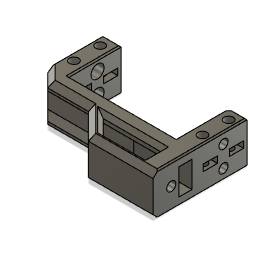
FrameAssembly v35 (Autodesk Fusion 360 archive; units mm, degrees)
design "FrameCenterServoHolder"
Autodesk Fusion 360 part; units mm, degrees
(part 1 of 2)
sketch "Sketch1" plane through (0, 0, 0) normal (0, 1, 0) x (1, 0, 0)
  line L0 (0, 26) -> (7, 26)
  line L1 (7, 26) -> (7, 6)
  line L2 (7, 6) -> (48, 6)
  line L3 (48, 6) -> (48, 26)
  line L4 (48, 26) -> (55, 26)
  line L5 (55, 26) -> (55, -9.8)
  line L6 (55, -9.8) -> (30.3, -9.8)
  line L7 (30.3, -9.8) -> (20.5, 0)
  line L8 (20.5, 0) -> (0, 0)
  line L9 (0, 26) -> (0, 0)
  line L10 (0, 0) -> (0, 39.3629) construction
  dimension "d1" = 7
  dimension "d2" = 7
  dimension "d3" = 41
  dimension "d4" = 6
  dimension "d5" = 15.8
  dimension "d7" = 135
  dimension "d8" = 20
  dimension "d98" = 20.5
  constraint perpendicular L0 L1
  constraint perpendicular L1 L2
  constraint perpendicular L2 L3
  constraint perpendicular L1 L4
  constraint perpendicular L4 L5
  constraint perpendicular L5 L6
  constraint collinear L0 L4
  constraint coincident L9.end L8
  constraint coincident L8.end L9.end
  constraint perpendicular L8 L9
  constraint vertical L10
  constraint collinear L9 L10
  measures "d1" distance of L0.start L0.end
  measures "d2" distance of L3.end L4.end
  measures "d3" distance of L1 L3
  measures "d4" distance of L2 L8
  measures "d5" distance of L2 L6
  measures "d7" angle of L6 L7
  measures "d8" distance of L2 L4
  measures "d98" distance of L7.end L8.end
extrude "Extrude1" add sketch "Sketch1" along normal blind 16
sketch "Sketch2" plane through (0, 16, 0) normal (0, 1, 0) x (-1, 0, 0)
  line L0 (-7, -26) -> (0, -26)
  line L1 (0, -26) -> (0, 0)
  line L2 (0, 0) -> (-20.5, 0)
  line L3 (-20.5, 0) -> (-30.3, 9.8)
  line L4 (-30.3, 9.8) -> (-55, 9.8)
  line L5 (-55, 9.8) -> (-55, -26)
  line L6 (-55, -26) -> (-48, -26)
  line L7 (-48, -26) -> (-48, -6)
  line L8 (-48, -6) -> (-7, -6)
  line L9 (-7, -6) -> (-7, -26)
  line L10 (-3, -22) -> (-52, -22) construction
  line L11 (-52, -22) -> (-52, -12) construction
  line L12 (-52, -12) -> (-3, -12) construction
  line L13 (-3, -12) -> (-3, -22) construction
  circle A0 centre (-3, -22) radius 1.75
  circle A1 centre (-3, -12) radius 1.75
  circle A2 centre (-52, -22) radius 1.75
  circle A3 centre (-52, -12) radius 1.75
  dimension "d11" = 3.5
  dimension "d12" = 3.5
  dimension "d13" = 3.5
  dimension "d14" = 3.5
  dimension "d15" = 49
  dimension "d16" = 10
  dimension "d17" = 55
  dimension "d18" = 20
  dimension "d19" = 4
  dimension "d20" = 3
  constraint horizontal L10
  constraint vertical L11
  constraint horizontal L12
  constraint vertical L13
  constraint coincident L10.start L13.end
  constraint coincident L12.end L13.start
  constraint coincident L10.end L11.start
  constraint coincident L11.end L12.start
  measures "d11" diameter of A0
  measures "d12" diameter of A1
  measures "d13" diameter of A2
  measures "d14" diameter of A3
  measures "d15" distance of L10.start L10.end
  measures "d16" distance of L10.start L12.end
  measures "d17" distance of L1 L5
  measures "d18" distance of L6.end L7.end
  measures "d19" distance of L6 L10
  measures "d20" distance of L1 L13
extrude "Extrude2" cut sketch "Sketch2" against normal up to surface (16 mm away) contours A0 | A1 | A2 | A3
ref_plane "WorkPlane1" through (27.5, 8, -8.1) normal (0, 1, 0) x (0, 0, 1)
ref_plane "WorkPlane2" through (27.5, 8, -16) normal (0, 0, -1) x (-1, 0, 0)
ref_plane "WorkPlane3" through (27.5, 8, -16) normal (-1, 0, 0) x (0, 0, 1)
ref_plane "WorkPlane4" through (27.5, 8, -8.1) normal (0, 1, 0) x (0, 0, 1)
sketch "Sketch3" plane through (27.5, 8, -7.6) normal (0, 1, 0) x (1, 0, 0)
  circle A0 centre (-24.5, 4.4) radius 1.75
  circle A1 centre (24.5, 14.4) radius 1.75
  circle A2 centre (-24.5, 14.4) radius 1.75
  circle A3 centre (24.5, 4.4) radius 1.75
  line L0 (-20.5, 18.4) -> (-27.5, 18.4)
  line L1 (-27.5, 18.4) -> (-27.5, -7.6)
  line L2 (-27.5, -7.6) -> (-7, -7.6)
  line L3 (-7, -7.6) -> (2.8, -17.4)
  line L4 (2.8, -17.4) -> (27.5, -17.4)
  line L5 (27.5, -17.4) -> (27.5, 18.4)
  line L6 (27.5, 18.4) -> (20.5, 18.4)
  line L7 (20.5, 18.4) -> (20.5, -1.6)
  line L8 (20.5, -1.6) -> (-20.5, -1.6)
  line L9 (-20.5, -1.6) -> (-20.5, 18.4)
  line L10 (-27.6177, 4.4) -> (-26.0588, 1.7)
  line L11 (-26.0588, 1.7) -> (-22.9412, 1.7)
  line L12 (-22.9412, 1.7) -> (-21.3823, 4.4)
  line L13 (-21.3823, 4.4) -> (-22.9412, 7.1)
  line L14 (-22.9412, 7.1) -> (-26.0588, 7.1)
  line L15 (-26.0588, 7.1) -> (-27.6177, 4.4)
  line L16 (-22.9412, 1.7) -> (-20.5, 1.7)
  line L17 (-26.0588, 1.7) -> (-27.5, 1.7)
  line L18 (-22.9412, 7.1) -> (-20.5, 7.1)
  line L19 (-26.0588, 7.1) -> (-27.5, 7.1)
  line L20 (-21.3823, 14.4) -> (-22.9412, 17.1)
  line L21 (-22.9412, 17.1) -> (-26.0588, 17.1)
  line L22 (-26.0588, 17.1) -> (-27.6177, 14.4)
  line L23 (-27.6177, 14.4) -> (-26.0588, 11.7)
  line L24 (-26.0588, 11.7) -> (-22.9412, 11.7)
  line L25 (-22.9412, 11.7) -> (-21.3823, 14.4)
  line L26 (-26.0588, 17.1) -> (-27.5, 17.1)
  line L27 (-26.0588, 11.7) -> (-27.5, 11.7)
  line L28 (-22.9412, 11.7) -> (-20.5, 11.7)
  line L29 (-22.9412, 17.1) -> (-20.5, 17.1)
  point P0 (-24.5, 4.4)
  point P1 (-24.5, 14.4)
  dimension "d23" = 5.4
  dimension "d88" = 5.4
  constraint coincident P0 A0.centre
  constraint parallel L2 L11
  constraint coincident L9 L16.end
  constraint perpendicular L9 L16
  constraint coincident L1 L17.end
  constraint perpendicular L1 L17
  constraint coincident L9 L18.end
  constraint perpendicular L9 L18
  constraint coincident L1 L19.end
  constraint perpendicular L1 L19
  constraint coincident P1 A2.centre
  constraint parallel L0 L21
  constraint coincident L1 L26.end
  constraint perpendicular L1 L26
  constraint coincident L1 L27.end
  constraint perpendicular L1 L27
  constraint coincident L9 L28.end
  constraint perpendicular L9 L28
  constraint coincident L9 L29.end
  constraint perpendicular L9 L29
  measures "d23" distance of L11 L14
  measures "d88" distance of L21 L24
extrude "Extrude3" cut sketch "Sketch3" along normal mid plane 2.5 contours L9 L20 L25 L28 L29 | L1 L22 L26 | L1 L20 L21 L22 L23 L24 L25 | L9 L12 L13 L16 L18 | L1 L23 L27 | L1 L10 L11 L12 L13 L14 L15 | L1 L15 L19 | L1 L10 L17
mirror "Mirror2" about plane through (27.5, 8, -16) normal (-1, 0, 0) of "Extrude3"
sketch "Sketch4" plane through (0, 16, 0) normal (0, 1, 0) x (-1, 0, 0)
  circle A0 centre (-3, -12) radius 1.75
  circle A1 centre (-52, -22) radius 1.75
  circle A2 centre (-3, -22) radius 1.75
  circle A3 centre (-52, -12) radius 1.75
  line L0 (-7, -26) -> (0, -26)
  line L1 (0, -26) -> (0, 0)
  line L2 (0, 0) -> (-20.5, 0)
  line L3 (-20.5, 0) -> (-30.3, 9.8)
  line L4 (-30.3, 9.8) -> (-55, 9.8)
  line L5 (-55, 9.8) -> (-55, -26)
  line L6 (-55, -26) -> (-48, -26)
  line L7 (-48, -26) -> (-48, -6)
  line L8 (-48, -6) -> (-7, -6)
  line L9 (-7, -6) -> (-7, -26)
  line L10 (-26.1569, 0) -> (-48, 0)
  line L11 (-48, 0) -> (-48, 5.8)
  line L12 (-48, 5.8) -> (-31.9569, 5.8)
  line L13 (-31.9569, 5.8) -> (-26.1569, 0)
  dimension "d30" = 4
  dimension "d31" = 4
  constraint parallel L2 L10
  constraint perpendicular L2 L11
  constraint perpendicular L11 L12
  constraint parallel L3 L13
  constraint collinear L2 L10
  constraint collinear L7 L11
  measures "d30" distance of L4 L12
  measures "d31" distance of L3 L13
extrude "Extrude4" cut sketch "Sketch4" against normal blind 16 contours L10 L11 L12 L13
sketch "Sketch5" plane through (55, 0, 0) normal (1, 0, 0) x (0, 0, -1)
  line L0 (14.7, 6.75) -> (9.3, 6.75)
  line L1 (9.3, 6.75) -> (9.3, 9.25)
  line L2 (9.3, 9.25) -> (14.7, 9.25)
  line L3 (14.7, 9.25) -> (14.7, 6.75)
  line L4 (-9.8, 0) -> (26, 0)
  line L5 (26, 0) -> (26, 16)
  line L6 (26, 16) -> (-9.8, 16)
  line L7 (-9.8, 16) -> (-9.8, 0)
  line L8 (-5.8, 16) -> (0, 16)
  line L9 (0, 16) -> (0, 0)
  line L10 (0, 0) -> (-5.8, 0)
  line L11 (-5.8, 0) -> (-5.8, 16)
  line L12 (10.25, 16) -> (13.75, 16)
  line L13 (10.25, 9.25) -> (13.75, 9.25)
  line L14 (20.25, 16) -> (23.75, 16)
  line L15 (13.75, 6.75) -> (10.25, 6.75)
  line L16 (13.75, 0) -> (10.25, 0)
  line L17 (23.75, 0) -> (20.25, 0)
  line L18 (6, 0) -> (6, 16)
  line L19 (6, 16) -> (6, 0)
  line L20 (-9.8, 8) -> (26, 8) construction
  circle A0 centre (-2.9, 8) radius 1.75
  line L21 (17, 16) -> (17, 0) construction
  circle A1 centre (17, 12) radius 1.75
  circle A2 centre (17, 4) radius 1.75
  line L22 (24.7, 6.75) -> (19.3, 6.75)
  line L23 (19.3, 6.75) -> (19.3, 9.25)
  line L24 (19.3, 9.25) -> (24.7, 9.25)
  line L25 (24.7, 9.25) -> (24.7, 6.75)
  line L26 (20.25, 9.25) -> (23.75, 9.25)
  line L27 (23.75, 6.75) -> (20.25, 6.75)
  line L28 (12, 16) -> (12, 0) construction
  line L29 (22, 16) -> (22, 0) construction
  dimension "d34" = 3.5
  dimension "d35" = 5.8
  dimension "d36" = 2.9
  dimension "d37" = 20
  dimension "d39" = 3.5
  dimension "d40" = 3.5
  dimension "d41" = 16
  dimension "d42" = 4
  dimension "d43" = 4
  dimension "d90" = 10
  dimension "d91" = 5
  constraint midpoint L7 L20.start
  constraint midpoint L5 L20.end
  constraint coincident L20 A0.centre
  constraint coincident L6 L21.start
  constraint coincident L4 L21.end
  constraint perpendicular L4 L21
  constraint coincident L21 A1.centre
  constraint coincident L21 A2.centre
  constraint midpoint L12 L28.start
  constraint midpoint L16 L28.end
  constraint midpoint L14 L29.start
  constraint midpoint L17 L29.end
  measures "d34" diameter of A0
  measures "d35" distance of L9 L11
  measures "d36" distance of L11 A0.centre
  measures "d37" distance of L5 L18
  measures "d39" diameter of A1
  measures "d40" diameter of A2
  measures "d41" distance of L4.end L5.end
  measures "d42" distance of L6 A1.centre
  measures "d43" distance of L4 A2.centre
  measures "d90" distance of L28 L29
  measures "d91" distance of L21 L28
extrude "Extrude5" cut sketch "Sketch5" against normal up to surface (7 mm away) contours A0 | A1 | A2
sketch "Sketch6" plane through (48, 0, 0) normal (-1, 0, 0) x (0, 0, 1)
  circle A0 centre (-17, 12) radius 1.75
  circle A1 centre (-17, 4) radius 1.75
  line L0 (-9.3, 6.75) -> (-14.7, 6.75)
  line L1 (-14.7, 6.75) -> (-14.7, 9.25)
  line L2 (-14.7, 9.25) -> (-9.3, 9.25)
  line L3 (-9.3, 9.25) -> (-9.3, 6.75)
  line L4 (-26, 0) -> (-6, 0)
  line L5 (-6, 0) -> (-6, 16)
  line L6 (-6, 16) -> (-26, 16)
  line L7 (-26, 16) -> (-26, 0)
  circle A2 centre (-17, 4) radius 2.9
  circle A3 centre (-17, 12) radius 2.9
  line L8 (-19.3, 6.75) -> (-24.7, 6.75)
  line L9 (-24.7, 6.75) -> (-24.7, 9.25)
  line L10 (-24.7, 9.25) -> (-19.3, 9.25)
  line L11 (-19.3, 9.25) -> (-19.3, 6.75)
  circle A4 centre (2.9, 8) radius 1.75
  line L12 (5.8, 16) -> (0, 16)
  line L13 (0, 16) -> (0, 0)
  line L14 (0, 0) -> (5.8, 0)
  line L15 (5.8, 0) -> (5.8, 16)
  circle A5 centre (2.9, 8) radius 2.9
  dimension "d46" = 5.8
  dimension "d47" = 5.8
  dimension "d89" = 5.8
  constraint concentric A1 A2
  constraint concentric A0 A3
  constraint concentric A4 A5
  measures "d46" diameter of A2
  measures "d47" diameter of A3
  measures "d89" diameter of A5
extrude "Extrude6" cut sketch "Sketch6" against normal blind 3 contours A2 | A3 | A5
sketch "Sketch7" plane through (0, 0, 0) normal (-1, 0, 0) x (0, 0, 1)
  line L0 (-9.3, 6.75) -> (-14.7, 6.75)
  line L1 (-14.7, 6.75) -> (-14.7, 9.25)
  line L2 (-14.7, 9.25) -> (-9.3, 9.25)
  line L3 (-9.3, 9.25) -> (-9.3, 6.75)
  line L4 (-26, 0) -> (0, 0)
  line L5 (0, 0) -> (0, 16)
  line L6 (0, 16) -> (-26, 16)
  line L7 (-26, 16) -> (-26, 0)
  line L8 (0, 0) -> (9.8, 0)
  line L9 (9.8, 0) -> (9.8, 16)
  line L10 (9.8, 16) -> (0, 16)
  line L11 (0, 16) -> (0, 0)
  line L12 (0, 13) -> (5, 13)
  line L13 (5, 13) -> (5, 3)
  line L14 (5, 3) -> (0, 3)
  line L15 (0, 3) -> (0, 13)
  line L16 (-19.3, 6.75) -> (-24.7, 6.75)
  line L17 (-24.7, 6.75) -> (-24.7, 9.25)
  line L18 (-24.7, 9.25) -> (-19.3, 9.25)
  line L19 (-19.3, 9.25) -> (-19.3, 6.75)
  circle A0 centre (2.9, 8) radius 2.9
  circle A1 centre (2.9, 8) radius 1.75
  dimension "d50" = 5
  dimension "d51" = 10
  dimension "d52" = 16
  dimension "d53" = 3
  constraint horizontal L12
  constraint vertical L13
  constraint horizontal L14
  constraint vertical L15
  constraint coincident L5 L12.start
  measures "d50" distance of L13 L15
  measures "d51" distance of L12.end L13.end
  measures "d52" distance of L8.end L9.end
  measures "d53" distance of L10 L12
extrude "Extrude7" cut sketch "Sketch7" along normal up to surface contours L5 L11 L13 L14 L15 A0 | L5 L11 L12 L13 L15 A0 | L13 A0 | L13 A0 | A1 end surface through (31.9569, 16, 5.8) normal (0.707107, 0, -0.707107) offset 0
sketch "Sketch8" plane through (27.5, 8, -7.6) normal (0, 1, 0) x (1, 0, 0)
  line L0 (20.5, -7.6) -> (20.5, -13.4)
  line L1 (20.5, -13.4) -> (4.4569, -13.4)
  circle A0 centre (-24.5, 4.4) radius 1.75
  circle A1 centre (24.5, 14.4) radius 1.75
  circle A2 centre (-24.5, 14.4) radius 1.75
  circle A3 centre (24.5, 4.4) radius 1.75
  line L2 (-20.5, 18.4) -> (-27.5, 18.4)
  line L3 (-27.5, 18.4) -> (-27.5, -7.6)
  line L4 (-1.3431, -7.6) -> (20.5, -7.6)
  line L5 (2.8, -17.4) -> (27.5, -17.4)
  line L6 (27.5, -17.4) -> (27.5, 18.4)
  line L7 (27.5, 18.4) -> (20.5, 18.4)
  line L8 (20.5, 18.4) -> (20.5, -1.6)
  line L9 (20.5, -1.6) -> (-20.5, -1.6)
  line L10 (-20.5, -1.6) -> (-20.5, 18.4)
  line L11 (20.5, -7.6) -> (27.5, -7.6)
  line L12 (27.5, -2.6) -> (13.5, -2.6)
  line L13 (13.5, -2.6) -> (4.8397, -7.6)
  line L14 (4.4569, -13.4) -> (-1.3431, -7.6)
  line L15 (-7, -7.6) -> (2.8, -17.4)
  line L16 (-27.5, -7.6) -> (-7, -7.6)
  dimension "d56" = 5
  dimension "d57" = 150
  dimension "d99" = 7
  dimension "d100" = 14
  constraint coincident L0.start L4.end
  constraint coincident L6 L11.end
  constraint perpendicular L6 L11
  constraint coincident L6 L12.start
  constraint perpendicular L6 L12
  constraint coincident L4 L13.end
  measures "d56" distance of L11 L12
  measures "d57" angle of L12 L13
  measures "d99" distance of L0.start L11.end
  measures "d100" distance of L12.start L12.end
extrude "Extrude8" cut sketch "Sketch8" along normal mid plane 10 contours L4 L6 L11 L12 L13
sketch "Sketch13" plane through (48, 0, 0) normal (-1, 0, 0) x (0, 0, 1)
  circle A0 centre (-17, 4) radius 2.9
  circle A1 centre (-17, 12) radius 2.9
  line L0 (-9.3, 6.75) -> (-14.7, 6.75)
  line L1 (-14.7, 6.75) -> (-14.7, 9.25)
  line L2 (-14.7, 9.25) -> (-9.3, 9.25)
  line L3 (-9.3, 9.25) -> (-9.3, 6.75)
  line L4 (-26, 0) -> (-6, 0)
  line L5 (-6, 0) -> (-6, 16)
  line L6 (-6, 16) -> (-26, 16)
  line L7 (-26, 16) -> (-26, 0)
  line L8 (-19.3, 6.75) -> (-24.7, 6.75)
  line L9 (-24.7, 6.75) -> (-24.7, 9.25)
  line L10 (-24.7, 9.25) -> (-19.3, 9.25)
  line L11 (-19.3, 9.25) -> (-19.3, 6.75)
  point P0 (-24, 16)
  point P1 (-26, 14)
  dimension "d81" = 2
  dimension "d82" = 2
  constraint coincident L6 P0
  constraint coincident L7 P1
  measures "d81" distance of L7 P0
  measures "d82" distance of L6 P1
sketch "Sketch14" plane through (0, 0, -26) normal (0, 0, -1) x (-1, 0, 0)
  line L0 (-55, 0) -> (-48, 0)
  line L1 (-48, 0) -> (-48, 16)
  line L2 (-48, 16) -> (-55, 16)
  line L3 (-55, 16) -> (-55, 0)
  point P0 (-50, 16)
  dimension "d83" = 2
  constraint coincident L2 P0
  measures "d83" distance of L1 P0
ref_plane "WorkPlane6" through (50, 16, -26) normal (0.57735, -0.57735, 0.57735) x (0.707107, 0.707107, 0)
sketch "Sketch15" plane through (50, 16, -26) normal (0.57735, -0.57735, 0.57735) x (0.712442, 0.701648, -0.010795)
  line L0 (-2.8282, -0.0374) -> (0, 0)
  line L1 (0, 0) -> (-1.4465, 2.4306)
  line L2 (-1.4465, 2.4306) -> (-2.8282, -0.0374)
  point P0 (-1.4465, 2.4306)
  point P1 (-2.8282, -0.0374)
  constraint coincident P1 L0.start
  constraint coincident L0.end L1.start
  constraint coincident P0 L1.end
extrude "Extrude11" cut sketch "Sketch15" against normal up to surface (1.1547 mm away)
mirror "Mirror4" about plane through (27.5, 8, -8.1) normal (0, 1, 0) of "Extrude11"
sketch "Sketch16" plane through (0, 0, 0) normal (-1, 0, 0) x (0, 0, 1)
  line L0 (-9.3, 6.75) -> (-14.7, 6.75)
  line L1 (-14.7, 6.75) -> (-14.7, 9.25)
  line L2 (-14.7, 9.25) -> (-9.3, 9.25)
  line L3 (-9.3, 9.25) -> (-9.3, 6.75)
  line L4 (-19.3, 6.75) -> (-24.7, 6.75)
  line L5 (-24.7, 6.75) -> (-24.7, 9.25)
  line L6 (-24.7, 9.25) -> (-19.3, 9.25)
  line L7 (-19.3, 9.25) -> (-19.3, 6.75)
  line L8 (-26, 0) -> (0, 0)
  line L9 (0, 0) -> (0, 16)
  line L10 (0, 16) -> (-26, 16)
  line L11 (-26, 16) -> (-26, 0)
  line L12 (0, 13) -> (5, 13)
  line L13 (5, 13) -> (5, 10)
  arc A0 (5, 6) -> (5, 10) centre (2.9, 8) ccw
  line L14 (5, 6) -> (5, 3)
  line L15 (5, 3) -> (0, 3)
  line L16 (0, 3) -> (0, 0)
  line L17 (0, 0) -> (9.8, 0)
  line L18 (9.8, 0) -> (9.8, 16)
  line L19 (9.8, 16) -> (0, 16)
  line L20 (0, 16) -> (0, 13)
  line L21 (0, 3) -> (-2, 5)
  line L22 (-2, 5) -> (-2, 11)
  line L23 (-2, 11) -> (0, 13)
  dimension "d93" = 45
  dimension "d94" = 45
  dimension "d95" = 2
  constraint coincident L15.end L16.start
  constraint perpendicular L15 L22
  constraint coincident L12.start L20.end
  measures "d93" angle of L9 L21
  measures "d94" angle of L9 L23
  measures "d95" distance of L9 L22
extrude "Extrude12" cut sketch "Sketch16" along normal up to surface contours L9 L21 L22 L23 end surface through (41, 8, -5) normal (0.5, 0, 0.866025) offset 0
sketch "Sketch9" plane through (0, 0, 0) normal (-1, 0, 0) x (0, 0, 1)
  line L0 (-26, 16) -> (-26, 0)
  line L1 (-9.3, 6.75) -> (-14.7, 6.75)
  line L2 (-14.7, 6.75) -> (-14.7, 9.25)
  line L3 (-14.7, 9.25) -> (-9.3, 9.25)
  line L4 (-9.3, 9.25) -> (-9.3, 6.75)
  line L5 (-9.3, 6.75) -> (-14.7, 6.75)
  line L6 (-14.7, 6.75) -> (-14.7, 9.25)
  line L7 (-14.7, 9.25) -> (-9.3, 9.25)
  line L8 (-9.3, 9.25) -> (-9.3, 6.75)
  circle A0 centre (-17, 12) radius 2.9
  circle A1 centre (-17, 4) radius 2.9
  line L9 (-6, 0) -> (-6, 16)
  circle A2 centre (-17, 12) radius 1.75
  circle A3 centre (-17, 4) radius 1.75
  circle A4 centre (-17, 12) radius 2.5
  circle A5 centre (-17, 4) radius 2.5
  line L10 (-24, 16) -> (-26, 14)
  line L11 (-26, 2) -> (-24, 0)
  line L12 (-24.7, 6.75) -> (-24.7, 9.25)
  line L13 (-19.3, 9.25) -> (-19.3, 6.75)
  line L14 (-24.7, 6.75) -> (-24.7, 9.25)
  line L15 (-19.3, 9.25) -> (-19.3, 6.75)
  line L16 (-19.3, 6.75) -> (-24.7, 6.75)
  line L17 (-24.7, 9.25) -> (-19.3, 9.25)
  line L18 (0, 3) -> (-2, 5)
  line L19 (-2, 5) -> (-2, 11)
  line L20 (-2, 11) -> (0, 13)
  line L21 (0, 13) -> (0, 16)
  line L22 (0, 16) -> (-26, 16)
  line L23 (-26, 0) -> (0, 0)
  line L24 (0, 0) -> (0, 3)
  line L25 (-24, 0) -> (-6, 0)
  line L26 (-6, 16) -> (-24, 16)
  line L27 (-26, 14) -> (-26, 2)
  line L28 (-19.3, 6.75) -> (-24.7, 6.75)
  line L29 (-24.7, 9.25) -> (-19.3, 9.25)
  dimension "d67" = 5
  dimension "d68" = 5
  constraint concentric A2 A4
  constraint concentric A3 A5
  measures "d67" diameter of A4
  measures "d68" diameter of A5
extrude "Extrude9" cut sketch "Sketch9" against normal up to surface (7 mm away) contours A2 | A3 | A4 | A5
chamfer "Chamfer1" distance 5 angle 45 2 edges at (0, 14.5, 0) (0, 1.5, 0)
chamfer "Chamfer5" distance 0.5 angle 45 4 edges at (48, 0, 2.9) (39.9784, 0, 5.8) (29.0569, 0, 2.9) (37.0784, 0, 0)
chamfer "Chamfer6" distance 1.5 angle 45 4 edges at (48, 16, 2.9) (39.9784, 16, 5.8) (29.0569, 16, 2.9) (37.0784, 16, 0)
chamfer "Chamfer7" distance 2 angle 45 8 edges at (2.5, 0, -2.5) (12.75, 0, 0) (25.4, 0, 4.9) (42.65, 0, 9.8) (42.65, 16, 9.8) (25.4, 16, 4.9) (12.75, 16, 0) (2.5, 16, -2.5)
chamfer "Chamfer8" distance 0.5 angle 45 7 edges at (55, 16, -9.1) (52.5, 16, -26) (48, 16, -15) (27.5, 16, -6) (7, 16, -16) (3.5, 16, -26) (0, 16, -16.9142)
chamfer "Chamfer8" distance 0.5 angle 45 1 edges at (48, 8, -26)
chamfer "Chamfer9" distance 0.5 angle 45 7 edges at (0, 0, -16.9142) (3.5, 0, -26) (7, 0, -16) (27.5, 0, -6) (48, 0, -16) (51.5, 0, -26) (55, 0, -9.1)
equation "d2 = d1"
equation "d12 = d11"
equation "d13 = d11"
equation "d14 = d11"
equation "d19 = ( d18 - d16 ) / 2 - 1 mm"
equation "d20 = ( d17 - d15 ) / 2"
equation "d31 = d30"
equation "d36 = d35 / 2"
equation "d39 = d34"
equation "d40 = d34"
equation "d42 = d41 / 4"
equation "d43 = d42"
equation "d47 = d46"
equation "d53 = ( d52 - d51 ) / 2"
equation "d68 = d67"
equation "d82 = d81"
equation "d88 = d23"
equation "d89 = d46"
equation "d91 = d90 / 2"
equation "d94 = d93"
equation "d100 = d99 * 2"

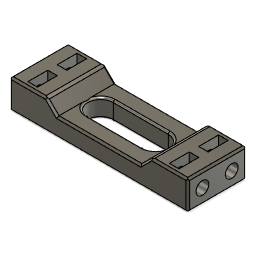
design "LegRib"
Autodesk Fusion 360 part; units mm, degrees
sketch "Sketch1" plane through (0, 0, 0) normal (0, 1, 0) x (1, 0, 0)
  line L0 (0, 0) -> (48.6, 0)
  line L1 (48.6, 0) -> (48.6, 16)
  line L2 (48.6, 16) -> (0, 16)
  line L3 (0, 16) -> (0, 0)
  dimension "d1" = 48.6
  dimension "d2" = 16
  constraint horizontal L0
  constraint vertical L1
  constraint horizontal L2
  constraint vertical L3
  constraint coincident L0.start L3.end
  measures "d1" distance of L1.end L2.end
  measures "d2" distance of L0.start L2.end
extrude "Extrude1" add sketch "Sketch1" along normal blind 8
sketch "Sketch2" plane through (0, 0, 0) normal (-1, 0, 0) x (0, 0, 1)
  line L0 (-16, 0) -> (0, 0)
  line L1 (0, 0) -> (0, 8)
  line L2 (0, 8) -> (-16, 8)
  line L3 (-16, 8) -> (-16, 0)
  line L4 (-16, 4) -> (0, 4) construction
  circle A0 centre (-12, 4) radius 1.75
  circle A1 centre (-4, 4) radius 1.75
  dimension "d5" = 3.5
  dimension "d6" = 3.5
  dimension "d7" = 16
  dimension "d8" = 4
  dimension "d9" = 4
  constraint midpoint L3 L4.start
  constraint midpoint L1 L4.end
  constraint coincident L4 A0.centre
  constraint coincident L4 A1.centre
  measures "d5" diameter of A0
  measures "d6" diameter of A1
  measures "d7" distance of L1.end L2.end
  measures "d8" distance of L3 A0.centre
  measures "d9" distance of L1 A1.centre
extrude "Extrude2" cut sketch "Sketch2" against normal blind 12 contours A0 | A1
ref_plane "WorkPlane1" through (5, 4, -8) normal (-1, 0, 0) x (0, 0, 1)
sketch "Sketch3" plane through (5, 4, -8) normal (-1, 0, 0) x (0, 0, -1)
  circle A0 centre (4, 0) radius 1.75
  circle A1 centre (-4, 0) radius 1.75
  line L0 (8, 4) -> (-8, 4)
  line L1 (-8, 4) -> (-8, -4)
  line L2 (-8, -4) -> (8, -4)
  line L3 (8, -4) -> (8, 4)
  line L4 (1.3, 1.5588) -> (1.3, -1.5588)
  line L5 (1.3, -1.5588) -> (4, -3.1177)
  line L6 (4, -3.1177) -> (6.7, -1.5588)
  line L7 (6.7, -1.5588) -> (6.7, 1.5588)
  line L8 (6.7, 1.5588) -> (4, 3.1177)
  line L9 (4, 3.1177) -> (1.3, 1.5588)
  line L10 (6.7, 4) -> (1.3, 4)
  line L11 (1.3, 4) -> (1.3, -4)
  line L12 (1.3, -4) -> (6.7, -4)
  line L13 (6.7, -4) -> (6.7, 4)
  point P0 (4, 0)
  dimension "d13" = 5.4
  constraint coincident P0 A0.centre
  constraint parallel L3 L7
  constraint horizontal L10
  constraint vertical L11
  constraint horizontal L12
  constraint vertical L13
  constraint coincident L2 L11.end
  constraint coincident L0 L10.start
  constraint collinear L7 L13
  constraint collinear L4 L11
  measures "d13" distance of L4 L7
extrude "Extrude3" cut sketch "Sketch3" along normal mid plane 2.6 contours L0 L8 L9 L10 L11 L13 | L4 L5 L6 L7 L8 L9 L11 L13 | L2 L5 L6 L11 L12 L13
ref_plane "WorkPlane2" through (24.3, 4, -8) normal (0, 0, -1) x (-1, 0, 0)
ref_plane "WorkPlane3" through (24.3, 4, -8) normal (-1, 0, 0) x (0, 0, 1)
mirror "Mirror1" about plane through (24.3, 4, -8) normal (0, 0, -1) of "Extrude3"
mirror "Mirror2" about plane through (24.3, 4, -8) normal (-1, 0, 0) of "Extrude2", "Extrude3", "Mirror1"
sketch "Sketch4" plane through (0, 0, 0) normal (0, 0, 1) x (1, 0, 0)
  line L0 (0, 0) -> (48.6, 0)
  line L1 (48.6, 0) -> (48.6, 8)
  line L2 (48.6, 8) -> (0, 8)
  line L3 (0, 8) -> (0, 0)
  line L4 (10, 8) -> (13, 5)
  line L5 (13, 5) -> (35.6, 5)
  line L6 (35.6, 5) -> (38.6, 8)
  dimension "d22" = 10
  dimension "d23" = 10
  dimension "d24" = 135
  dimension "d25" = 135
  dimension "d26" = 3
  constraint coincident L2 L4.start
  constraint parallel L2 L5
  constraint coincident L2 L6.end
  measures "d22" distance of L3 L4.start
  measures "d23" distance of L1 L6.end
  measures "d24" angle of L4 L5
  measures "d25" angle of L5 L6
  measures "d26" distance of L2 L5
extrude "Extrude4" cut sketch "Sketch4" against normal blind 16 contours L2 L4 L5 L6
sketch "Sketch5" plane through (0, 0, 0) normal (0, -1, 0) x (1, 0, 0)
  line L0 (42.3, -6.7) -> (42.3, -1.3)
  line L1 (42.3, -1.3) -> (44.9, -1.3)
  line L2 (44.9, -1.3) -> (44.9, -6.7)
  line L3 (44.9, -6.7) -> (42.3, -6.7)
  line L4 (42.3, -14.7) -> (42.3, -9.3)
  line L5 (42.3, -9.3) -> (44.9, -9.3)
  line L6 (44.9, -9.3) -> (44.9, -14.7)
  line L7 (44.9, -14.7) -> (42.3, -14.7)
  line L8 (6.3, -1.3) -> (6.3, -6.7)
  line L9 (6.3, -6.7) -> (3.7, -6.7)
  line L10 (3.7, -6.7) -> (3.7, -1.3)
  line L11 (3.7, -1.3) -> (6.3, -1.3)
  line L12 (6.3, -9.3) -> (6.3, -14.7)
  line L13 (6.3, -14.7) -> (3.7, -14.7)
  line L14 (3.7, -14.7) -> (3.7, -9.3)
  line L15 (3.7, -9.3) -> (6.3, -9.3)
  line L16 (0, 0) -> (0, -16)
  line L17 (0, -16) -> (48.6, -16)
  line L18 (48.6, -16) -> (48.6, 0)
  line L19 (48.6, 0) -> (0, 0)
  line L20 (0, -8) -> (48.6, -8) construction
  line L21 (16.8, -11.5) -> (31.8, -11.5)
  arc A0 (31.8, -11.5) -> (31.8, -4.5) centre (31.8, -8) ccw
  line L22 (31.8, -4.5) -> (16.8, -4.5)
  arc A1 (16.8, -4.5) -> (16.8, -11.5) centre (16.8, -8) ccw
  line L23 (16.8, -8) -> (31.8, -8) construction
  dimension "d29" = 7
  dimension "d30" = 15
  dimension "d31" = 48.6
  dimension "d32" = 16.8
  constraint midpoint L16 L20.start
  constraint midpoint L18 L20.end
  constraint tangent L21 A0
  constraint tangent A0 L22
  constraint parallel L21 L22
  constraint tangent L22 A1
  constraint tangent L21 A1
  constraint coincident L20 A0.centre
  constraint parallel L20 L23
  measures "d29" distance of L21 L22
  measures "d30" distance of A1.centre A0.centre
  measures "d31" distance of L16.start L18.end
  measures "d32" distance of L16 A1.centre
extrude "Extrude5" cut sketch "Sketch5" against normal up to surface (8 mm away) contours L21 A0 L22 A1
chamfer "Chamfer1" distance 0.5 angle 45 10 edges at (48.6, 8, -8) (5, 8, 0) (43.6, 8, 0) (0, 8, -8) (5, 8, -16) (43.6, 8, -16) (24.3, 0, -16) (48.6, 0, -8) (24.3, 0, 0) (0, 0, -8)
chamfer "Chamfer3" distance 0.5 angle 45 4 edges at (0, 4, -16) (0, 4, 0) (48.6, 4, 0) (48.6, 4, -16)
chamfer "Chamfer4" distance 0.5 angle 45 8 edges at (11.75, 6.25, 0) (24.3, 5, 0) (36.85, 6.25, 0) (38.6, 8, -8) (36.85, 6.25, -16) (24.3, 5, -16) (11.75, 6.25, -16) (10, 8, -8)
fillet "Fillet1" radius 0.5 4 edges at (13.3, 5, -8) (24.3, 5, -11.5) (35.3, 5, -8) (24.3, 5, -4.5)
fillet "Fillet2" radius 0.5 4 edges at (24.3, 0, -11.5) (13.3, 0, -8) (24.3, 0, -4.5) (35.3, 0, -8)
equation "d6 = d5"
equation "d8 = d7 / 4"
equation "d9 = d8"
equation "d23 = d22"
equation "d25 = d24"
equation "d32 = ( d31 - d30 ) / 2"

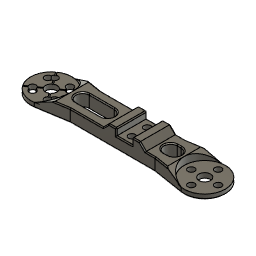
design "FemurSide2"
Autodesk Fusion 360 part; units mm, degrees
sketch "Sketch1" plane through (0, 0, 0) normal (0, 1, 0) x (1, 0, 0)
  line L0 (0, 0) -> (92, 0)
  line L1 (92, 0) -> (92, 16)
  line L2 (92, 16) -> (0, 16)
  line L3 (0, 16) -> (0, 0)
  dimension "d1" = 16
  dimension "d2" = 92
  constraint horizontal L0
  constraint vertical L1
  constraint horizontal L2
  constraint vertical L3
  constraint coincident L0.start L3.end
  measures "d1" distance of L0.start L2.end
  measures "d2" distance of L1.end L2.end
extrude "Extrude1" add sketch "Sketch1" along normal blind 6.5
ref_plane "WorkPlane1" through (46, 3.25, -8) normal (0, 0, 1) x (1, 0, 0)
ref_plane "WorkPlane2" through (46, 3.25, -8) normal (1, 0, 0) x (0, 0, -1)
sketch "Sketch2" plane through (0, 0, 0) normal (0, -1, 0) x (1, 0, 0)
  line L0 (0, 0) -> (0, -16)
  line L1 (0, -16) -> (92, -16)
  line L2 (92, -16) -> (92, 0)
  line L3 (92, 0) -> (0, 0)
  line L4 (0, -8) -> (92, -8) construction
  circle A0 centre (6, -8) radius 10.75
  line L5 (23.901, 0) -> (23.901, -16) construction
  dimension "d5" = 6
  dimension "d6" = 21.5
  dimension "d21" = 23.901
  constraint midpoint L0 L4.start
  constraint midpoint L2 L4.end
  constraint coincident L4 A0.centre
  constraint coincident L3 L5.start
  constraint coincident L1 L5.end
  constraint perpendicular L1 L5
  measures "d5" distance of L0 A0.centre
  measures "d6" diameter of A0
  measures "d21" distance of L0.end L5
extrude "Extrude2" add sketch "Sketch2" against normal up to surface (6.5 mm away) contours L0 L1 L3 A0 picked at (-1.5735, -7.7341)
sketch "Sketch3" plane through (0, 6.5, 0) normal (0, 1, 0) x (-1, 0, 0)
  line L0 (-13.1807, 0) -> (-92, 0)
  line L1 (-92, 0) -> (-92, -16)
  line L2 (-92, -16) -> (-13.1807, -16)
  arc A0 (-13.1807, -16) -> (-13.1807, 0) centre (-6, -8) ccw
  circle A1 centre (-6, -8) radius 3
  dimension "d9" = 6
  constraint concentric A0 A1
  measures "d9" diameter of A1
extrude "Extrude3" cut sketch "Sketch3" against normal blind 6.5 contours A1
sketch "Sketch4" plane through (0, 6.5, 0) normal (0, 1, 0) x (-1, 0, 0)
  circle A0 centre (-6, -8) radius 3
  line L0 (-13.1807, 0) -> (-92, 0)
  line L1 (-92, 0) -> (-92, -16)
  line L2 (-92, -16) -> (-13.1807, -16)
  arc A1 (-13.1807, -16) -> (-13.1807, 0) centre (-6, -8) ccw
  circle A2 centre (-6, -8) radius 10.75
  constraint concentric A0 A2
  constraint coincident L0.start A2
extrude "Extrude4" cut sketch "Sketch4" against normal up to surface (4 mm away) contours A1 A2
sketch "Sketch6" plane through (0, 0, 0) normal (0, -1, 0) x (1, 0, 0)
  circle A0 centre (6, -8) radius 3
  line L0 (13.1807, -16) -> (92, -16)
  line L1 (92, -16) -> (92, 0)
  line L2 (92, 0) -> (13.1807, 0)
  arc A1 (13.1807, 0) -> (13.1807, -16) centre (6, -8) ccw
  line L3 (0, 0) -> (92, 0)
  line L4 (0, -16) -> (0, 0)
  line L5 (92, -16) -> (0, -16)
  line L6 (23.901, 0) -> (23.901, -16) construction
  line L7 (7.7128, 2.6127) -> (23.901, 0)
  line L8 (7.7128, -18.6127) -> (23.901, -16)
  dimension "d22" = 23.901
  constraint coincident L3 L6.start
  constraint coincident L0 L6.end
  constraint perpendicular L0 L6
  constraint coincident A1 L7.start
  constraint coincident A1 L8.start
  constraint tangent A1 L7
  constraint tangent A1 L8
  measures "d22" distance of L4 L6
extrude "Extrude6" add sketch "Sketch6" against normal up to surface (6.5 mm away) contours L0 A1 L5 L8 | L2 A1 L3 L7
sketch "Sketch5" plane through (0, 2.5, 0) normal (0, 1, 0) x (-1, 0, 0)
  circle A0 centre (-6, -8) radius 3
  arc A1 (-7.7128, 2.6127) -> (-7.7128, -18.6127) centre (-6, -8) ccw
  arc A2 (-7.7128, -18.6127) -> (-7.7128, 2.6127) centre (-6, -8) ccw
  line L0 (-6, -8) -> (4.75, -8) construction
  line L1 (-6, -8) -> (2.8059, -1.8341) construction
  circle A3 centre (-6, -8) radius 7 construction
  circle A4 centre (-0.2659, -3.985) radius 1.75
  circle A5 centre (-10.015, -2.2659) radius 1.75
  circle A6 centre (-11.7341, -12.015) radius 1.75
  circle A7 centre (-1.985, -13.7341) radius 1.75
  line L2 (-6, -8) -> (2.8059, -14.1659) construction
  circle A8 centre (-0.2659, -12.015) radius 1.75
  circle A9 centre (-1.985, -2.2659) radius 1.75
  circle A10 centre (-11.7341, -3.985) radius 1.75
  circle A11 centre (-10.015, -13.7341) radius 1.75
  dimension "d60" = 35
  dimension "d61" = 3.5
  dimension "d62" = 14
  dimension "d64" = 360
  dimension "d65" = 35
  dimension "d66" = 3.5
  dimension "d68" = 360
  constraint coincident A0.centre A1.centre
  constraint midpoint A2 L0.end
  constraint coincident A2 L1.end
  constraint coincident A3 A4.centre
  constraint coincident L1 A4.centre
  constraint coincident A2 L2.end
  constraint coincident L2 A8.centre
  constraint coincident A3 A8.centre
  measures "d60" angle of L0 L1
  measures "d61" diameter of A4
  measures "d62" diameter of A3
  measures "d65" angle of L0 L2
  measures "d66" diameter of A8
extrude "Extrude5" cut sketch "Sketch5" against normal up to surface (2.5 mm away) contours A4 A9 | A4 A9 | A4 A9 | A5 A10 | A5 A10 | A5 A10 | A6 A11 | A6 A11 | A6 A11 | A7 A8 | A7 A8 | A7 A8
sketch "Sketch12" plane through (0, 2.5, 0) normal (0, 1, 0) x (-1, 0, 0)
  circle A0 centre (-6, -8) radius 3
  arc A1 (-7.7128, 2.6127) -> (-7.7128, -18.6127) centre (-6, -8) ccw
  arc A2 (-7.7128, -18.6127) -> (-7.7128, 2.6127) centre (-6, -8) ccw
  arc A3 (-9.9843, -4.0157) -> (-11.7648, -2.2352) centre (-10.015, -2.2659) ccw
  arc A4 (-11.7648, -2.2352) -> (-9.9843, -4.0157) centre (-11.7341, -3.985) ccw
  arc A5 (-11.7648, -13.7648) -> (-9.9843, -11.9843) centre (-10.015, -13.7341) ccw
  arc A6 (-9.9843, -11.9843) -> (-11.7648, -13.7648) centre (-11.7341, -12.015) ccw
  arc A7 (-2.0157, -4.0157) -> (-0.2352, -2.2352) centre (-0.2659, -3.985) ccw
  arc A8 (-0.2352, -2.2352) -> (-2.0157, -4.0157) centre (-1.985, -2.2659) ccw
  arc A9 (-0.2352, -13.7648) -> (-2.0157, -11.9843) centre (-0.2659, -12.015) ccw
  arc A10 (-2.0157, -11.9843) -> (-0.2352, -13.7648) centre (-1.985, -13.7341) ccw
  line L0 (-6, -8) -> (2.8059, -1.8341)
  constraint coincident A0.centre A1.centre
  constraint coincident A2 L0.end
  constraint coincident A7.centre L0
ref_plane "WorkPlane3" through (-2.8059, 2.5, -1.8341) normal (-0.819152, 0, 0.573576) x (0, -1, 0)
sketch "Sketch13" plane through (-2.8059, 2.5, -1.8341) normal (-0.819152, 0, 0.573576) x (0, -1, 0)
  line L0 (0, -7.711) -> (2.5, -7.711)
  line L1 (2.5, -10.75) -> (2.5, 9.6758)
  line L2 (2.5, 9.6758) -> (0, 9.6758)
  line L3 (0, -10.75) -> (0, 9.6758)
  line L4 (-4, 10.75) -> (-4, -7.711)
  line L5 (-4, -7.711) -> (0, -7.711)
  line L6 (0, -7.711) -> (0, 10.75)
  line L7 (0, 9.6758) -> (-4, 9.6758)
  circle A0 centre (0, 0) radius 0.3
  dimension "d69" = 0.6
  constraint coincident A0.centre origin
  measures "d69" diameter of A0
sweep "Sweep1" cut profiles "Sketch13" path "Sketch12" along L0 section 1 contours L3 L6 A0 | L3 L6 A0
pattern_circular "C-Pattern1" count 4 over 360 about axis through (6, -0.2489, -8) along (0, -1, 0) of "Sweep1"
sketch "Sketch7" plane through (46, 3.25, -8) normal (0, 0, 1) x (1, 0, 0)
  line L0 (-29.25, 3.25) -> (-38.2872, 3.25)
  line L1 (-38.2872, 3.25) -> (-38.2872, -0.75)
  line L2 (-38.2872, -0.75) -> (-34.0822, -0.75)
  line L3 (-38.2872, -0.75) -> (-38.2872, 3.25)
  line L4 (-38.5336, -0.75) -> (-42.2731, -0.75)
  line L5 (-38.2872, -0.75) -> (-34.0822, -0.75)
  line L6 (-48.6304, -0.75) -> (-38.2872, -0.75)
  line L7 (-22.099, 3.25) -> (-38.2872, 3.25)
  line L8 (-38.2872, 3.25) -> (-38.2872, -0.75)
  line L9 (-38.2872, -0.75) -> (-38.2872, -3.25)
  line L10 (-38.2872, -3.25) -> (-22.099, -3.25)
  line L11 (-22.099, -3.25) -> (-22.099, 3.25)
  line L12 (-29.25, 3.25) -> (-38.2872, -0.75)
  line L13 (-45.7648, -0.75) -> (-42.265, -0.75)
  line L14 (-37.735, -0.75) -> (-35.2418, -0.75)
  line L15 (-37.735, -0.75) -> (-34.2352, -0.75)
  line L16 (-44.7582, -0.75) -> (-42.265, -0.75)
  spline S0 degree 3 poles (-33.8341, -0.45) (-33.8649, -0.45) (-33.898, -0.4575) (-33.9589, -0.4881) (-33.9869, -0.5112) (-34.0311, -0.5645) (-34.0504, -0.5982) (-34.0759, -0.6721) (-34.0822, -0.7123) (-34.0822, -0.75) knots 0.045205 0.045205 0.045205 0.045205 0.056506 0.056506 0.067807 0.067807 0.079109 0.079109 0.09041 0.09041 0.09041 0.09041
  line L17 (-38.2872, -0.75) -> (-31.3696, -0.75)
  spline S1 degree 3 poles (-31.3696, -0.75) (-31.3696, -0.7123) (-31.3651, -0.6721) (-31.3469, -0.5982) (-31.3332, -0.5645) (-31.3018, -0.5112) (-31.282, -0.4881) (-31.2389, -0.4575) (-31.2157, -0.45) (-31.1941, -0.45) knots 0 0 0 0 0.011301 0.011301 0.022602 0.022602 0.033904 0.033904 0.045205 0.045205 0.045205 0.045205
  spline S2 degree 3 poles (-31.1941, -0.45) (-31.1725, -0.45) (-31.1496, -0.4575) (-31.1079, -0.4881) (-31.089, -0.5112) (-31.0593, -0.5645) (-31.0465, -0.5982) (-31.0296, -0.6721) (-31.0255, -0.7123) (-31.0255, -0.75) knots 0.045205 0.045205 0.045205 0.045205 0.056506 0.056506 0.067807 0.067807 0.079109 0.079109 0.09041 0.09041 0.09041 0.09041
  line L18 (-33.5907, -0.75) -> (-29.25, -0.75)
  spline S3 degree 3 poles (-33.5907, -0.75) (-33.5907, -0.7123) (-33.5968, -0.6721) (-33.6214, -0.5982) (-33.64, -0.5645) (-33.683, -0.5112) (-33.7103, -0.4881) (-33.7704, -0.4575) (-33.8032, -0.45) (-33.8341, -0.45) knots 0 0 0 0 0.011301 0.011301 0.022602 0.022602 0.033904 0.033904 0.045205 0.045205 0.045205 0.045205
  line L19 (-37.2196, -0.75) -> (-38.5336, -0.75)
  line L20 (-42.2731, -0.75) -> (-44.1497, -0.75)
  line L21 (-44.1497, -0.75) -> (-43.9843, -0.75)
  line L22 (-46.9743, -0.75) -> (-45.7648, -0.75)
  line L23 (-46.9743, -0.75) -> (-48.6304, -0.75)
  line L24 (-34.0822, -0.75) -> (-35.2418, -0.75)
  line L25 (-37.7269, -0.75) -> (-35.8503, -0.75)
  line L26 (-36.0157, -0.75) -> (-35.8503, -0.75)
  line L27 (-34.2352, -0.75) -> (-33.0257, -0.75)
  line L28 (-33.0257, -0.75) -> (-31.3696, -0.75)
  line L29 (-38.2872, -0.75) -> (-31.3696, -0.75)
  line L30 (-45.9178, -0.75) -> (-38.2872, -0.75)
  line L31 (-45.9178, -0.75) -> (-44.7582, -0.75)
  line L32 (-42.7804, -0.75) -> (-41.4664, -0.75)
  line L33 (-37.7269, -0.75) -> (-41.4664, -0.75)
  constraint coincident L0.start L12.start
  constraint coincident L1.end L2.start
extrude "Extrude7" cut sketch "Sketch7" along normal through all and the other way through all contours L0 L1 L3 L7 L8 L12
mirror "Mirror1" about plane through (46, 3.25, -8) normal (1, 0, 0) of "Extrude2", "Extrude3", "Extrude4", "Extrude6", "Extrude7"
sketch "Sketch14" plane through (0, 2.5, 0) normal (0, 1, 0) x (-1, 0, 0)
  circle A0 centre (-86, -8) radius 3
  arc A1 (-84.2872, -18.6127) -> (-84.2872, 2.6127) centre (-86, -8) ccw
  arc A2 (-84.2872, 2.6127) -> (-84.2872, -18.6127) centre (-86, -8) ccw
  line L0 (-86, -8) -> (-96.75, -8) construction
  circle A3 centre (-86, -8) radius 7 construction
  circle A4 centre (-93, -8) radius 1.75
  circle A5 centre (-86, -15) radius 1.75
  circle A6 centre (-79, -8) radius 1.75
  circle A7 centre (-86, -1) radius 1.75
  dimension "d78" = 14
  dimension "d79" = 3.5
  dimension "d81" = 360
  constraint coincident A0.centre A1.centre
  constraint midpoint A2 L0.end
  constraint concentric A0 A3
  constraint coincident A3 A4.centre
  constraint coincident L0 A4.centre
  measures "d78" diameter of A3
  measures "d79" diameter of A4
extrude "Extrude12" cut sketch "Sketch14" against normal up to surface (2.5 mm away) contours A4 | A5 | A6 | A7
sketch "Sketch8" plane through (0, 6.5, 0) normal (0, 1, 0) x (-1, 0, 0)
  line L0 (-75.25, -8) -> (-75.25, -17.1541)
  line L1 (-75.25, -17.1541) -> (-68.099, -16)
  line L2 (-68.099, -16) -> (-23.901, -16)
  line L3 (-23.901, -16) -> (-16.75, -17.1541)
  line L4 (-16.75, -17.1541) -> (-16.75, -8)
  line L5 (-16.75, -8) -> (-16.75, 1.1541)
  line L6 (-16.75, 1.1541) -> (-23.901, 0)
  line L7 (-23.901, 0) -> (-68.099, 0)
  line L8 (-68.099, 0) -> (-75.25, 1.1541)
  line L9 (-75.25, 1.1541) -> (-75.25, -8)
  arc A0 (-84.2872, -18.6127) -> (-84.2872, 2.6127) centre (-86, -8) ccw
  arc A1 (-84.2872, 2.6127) -> (-84.2872, -18.6127) centre (-86, -8) ccw
  circle A2 centre (-86, -8) radius 3
  arc A3 (-84.2872, -18.6127) -> (-75.25, -8) centre (-86, -8) ccw
  line L10 (-84.2872, -18.6127) -> (-75.25, -17.1541)
  line L11 (-75.25, -17.1541) -> (-75.25, -8)
  arc A4 (-75.25, -8) -> (-84.2872, 2.6127) centre (-86, -8) ccw
  line L12 (-75.25, -8) -> (-75.25, 1.1541)
  line L13 (-75.25, 1.1541) -> (-84.2872, 2.6127)
  arc A5 (2.6304, -1.5907) -> (-7.7128, 2.6127) centre (-6, -8) ccw
  arc A6 (-7.7128, 2.6127) -> (-11.9178, 0.9745) centre (-6, -8) ccw
  arc A7 (-16.75, -8) -> (-7.7128, -18.6127) centre (-6, -8) ccw
  line L14 (-16.75, -8) -> (-16.75, -17.1541)
  line L15 (-16.75, -17.1541) -> (-7.7128, -18.6127)
  arc A8 (-7.7128, 2.6127) -> (-16.75, -8) centre (-6, -8) ccw
  line L16 (-7.7128, 2.6127) -> (-16.75, 1.1541)
  line L17 (-16.75, 1.1541) -> (-16.75, -8)
  line L18 (-52, -16) -> (-52, 0) construction
  line L19 (-47.9, -16) -> (-47.9, 0)
  line L20 (-56.1, -16) -> (-56.1, 0)
  arc A9 (-3.2196, -12.4938) -> (-1.2418, -15.3184) centre (-1.985, -13.7341) ccw
  arc A10 (-3.7269, -6.0422) -> (-7.4664, -5.3828) centre (-6, -8) ccw
  arc A11 (-11.7648, -13.7648) -> (-9.9843, -11.9843) centre (-10.015, -13.7341) ccw
  arc A12 (-0.2352, -2.2352) -> (-2.0157, -4.0157) centre (-1.985, -2.2659) ccw
  arc A13 (-8.7804, -3.5062) -> (-10.7582, -0.6816) centre (-10.015, -2.2659) ccw
  circle A14 centre (-93, -8) radius 1.75
  circle A15 centre (-86, -1) radius 1.75
  circle A16 centre (-86, -15) radius 1.75
  circle A17 centre (-79, -8) radius 1.75
  line L21 (-8.7804, -3.5062) -> (-7.4664, -5.3828)
  line L22 (-3.7269, -6.0422) -> (-1.8503, -4.7281)
  arc A18 (-2.0157, -4.0157) -> (-1.8503, -4.7281) centre (-0.2659, -3.985) ccw
  arc A19 (0.9743, -2.7503) -> (-0.2352, -2.2352) centre (-0.2659, -3.985) ccw
  line L23 (0.9743, -2.7503) -> (2.6304, -1.5907)
  line L24 (-11.9178, 0.9745) -> (-10.7582, -0.6816)
  arc A20 (-7.7128, -18.6127) -> (-0.0822, -16.9745) centre (-6, -8) ccw
  line L25 (-0.0822, -16.9745) -> (-1.2418, -15.3184)
  line L26 (-3.2196, -12.4938) -> (-4.5336, -10.6172)
  arc A21 (-8.2731, -9.9578) -> (-4.5336, -10.6172) centre (-6, -8) ccw
  line L27 (-8.2731, -9.9578) -> (-10.1497, -11.2719)
  arc A22 (-9.9843, -11.9843) -> (-10.1497, -11.2719) centre (-11.7341, -12.015) ccw
  arc A23 (-12.9743, -13.2497) -> (-11.7648, -13.7648) centre (-11.7341, -12.015) ccw
  line L28 (-12.9743, -13.2497) -> (-14.6304, -14.4093)
  arc A24 (-14.6304, -14.4093) -> (-7.7128, -18.6127) centre (-6, -8) ccw
  dimension "d28" = 34
  dimension "d29" = 8.2
  dimension "d30" = 4.1
  constraint coincident L2 L18.start
  constraint coincident L7 L18.end
  constraint perpendicular L7 L18
  constraint coincident L2 L19.start
  constraint coincident L7 L19.end
  constraint perpendicular L7 L19
  constraint coincident L2 L20.start
  constraint coincident L7 L20.end
  constraint perpendicular L7 L20
  measures "d28" distance of A0.centre L18
  measures "d29" distance of L19 L20
  measures "d30" distance of L18 L19
extrude "Extrude8" cut sketch "Sketch8" against normal blind 0.5 contours L2 L7 L19 L20
sketch "Sketch9" plane through (0, 0, 0) normal (0, 0, 1) x (1, 0, 0)
  line L0 (47.9, 6) -> (47.9, 6.5)
  line L1 (47.9, 6.5) -> (23.901, 6.5)
  line L2 (23.901, 6.5) -> (23.901, 0)
  line L3 (23.901, 0) -> (68.099, 0)
  line L4 (68.099, 0) -> (68.099, 6.5)
  line L5 (68.099, 6.5) -> (56.1, 6.5)
  line L6 (56.1, 6.5) -> (56.1, 6)
  line L7 (56.1, 6) -> (47.9, 6)
  line L8 (47.9, 6.5) -> (43.9, 6.5)
  line L9 (43.9, 6.5) -> (43.9, 9.5)
  line L10 (43.9, 9.5) -> (47.9, 9.5)
  line L11 (47.9, 9.5) -> (47.9, 6.5)
  line L12 (52, 6) -> (52, 0) construction
  line L13 (60.1, 6.5) -> (60.1, 9.5)
  line L14 (60.1, 9.5) -> (56.1, 9.5)
  line L15 (56.1, 9.5) -> (56.1, 6.5)
  dimension "d33" = 4
  dimension "d34" = 3
  constraint horizontal L8
  constraint vertical L9
  constraint horizontal L10
  constraint vertical L11
  constraint coincident L0.end L1.start
  constraint midpoint L7 L12.start
  constraint coincident L3 L12.end
  constraint perpendicular L3 L12
  constraint symmetric L0.end L12 L5.end
  constraint symmetric L8.end L12 L13.start
  constraint symmetric L9.end L12 L13.end
  constraint symmetric L10.end L12 L14.end
  measures "d33" distance of L9.end L10.end
  measures "d34" distance of L8.end L9.end
extrude "Extrude9" add sketch "Sketch9" against normal up to surface (16 mm away) contours L1 L8 L9 L10 L11 | L5 L13 L14 L15
chamfer "Chamfer1" distance 3 angle 45 2 edges at (60.1, 6.5, -8) (43.9, 6.5, -8)
sketch "Sketch10" plane through (0, 6, 0) normal (0, 1, 0) x (-1, 0, 0)
  line L0 (-47.9, -16) -> (-47.9, 0)
  line L1 (-47.9, 0) -> (-56.1, 0)
  line L2 (-56.1, 0) -> (-56.1, -16)
  line L3 (-56.1, -16) -> (-47.9, -16)
  line L4 (-52, -16) -> (-52, 0) construction
  circle A0 centre (-52, -12) radius 1.75
  circle A1 centre (-52, -4) radius 1.75
  dimension "d38" = 3.5
  dimension "d39" = 3.5
  dimension "d40" = 8
  dimension "d41" = 4
  dimension "d42" = 16
  constraint midpoint L3 L4.start
  constraint midpoint L1 L4.end
  constraint coincident L4 A0.centre
  constraint coincident L4 A1.centre
  measures "d38" diameter of A0
  measures "d39" diameter of A1
  measures "d40" distance of A0.centre A1.centre
  measures "d41" distance of L3 A0.centre
  measures "d42" distance of L1.end L2.end
extrude "Extrude10" cut sketch "Sketch10" against normal up to surface (6 mm away) contours A0 | A1